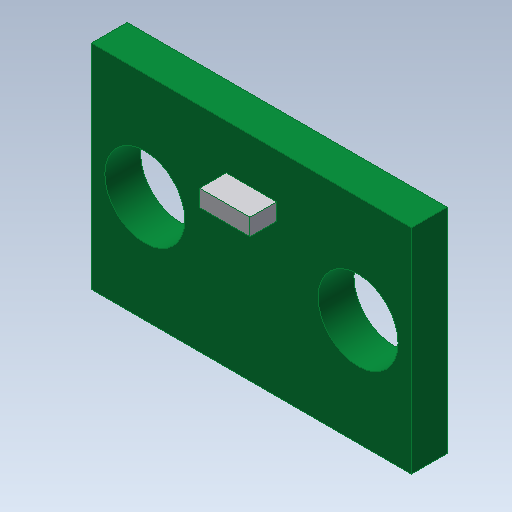
# Autodesk Inventor part: J002609
Saved by Autodesk Inventor 2020.3 (Build 243373000, 373)
## iProperties
RuleStatus: InUse
AfterDocSave0: file://Part Number Cleaner
Created: 2014-07-03
Material: Generic
Vendor: HHMI: JFRC - ID&F
Document SubType Name: Modeling
Designer: NEGRASHOVI
Density: 1 g/cm^3
Part Number: J002609
Appearance: Smooth - Dark Forest Green
DESIGN DEPARTMENT: HHMI: JFRC - ID&F
ALTERED ITEM PART NUMBER: N/A
ALTERED ITEM VENDOR: N/A
ALTERED ITEM DESCRIPTION: N/A
Author: NEGRASHOVI
Revision Number: 0
Autodesk Inventor part; units mm, degrees
ref_plane "YZ Plane" through (0, 0, 0) normal (1, 0, 0) x (0, 1, 0)
ref_plane "XZ Plane" through (0, 0, 0) normal (0, 1, 0) x (-1, 0, 0)
ref_plane "XY Plane" through (0, 0, 0) normal (0, 0, 1) x (1, 0, 0)
sketch "Sketch1" plane through (0, 0, 0) normal (0, 0, 1) x (1, 0, 0)
  line L0 (-7.62, -7.62) -> (7.62, -7.62)
  line L1 (7.62, -7.62) -> (7.62, 2.54)
  line L2 (7.62, 2.54) -> (-7.62, 2.54)
  line L3 (-7.62, 2.54) -> (-7.62, -7.62)
  line L4 (-10.668, 0) -> (10.668, 0) construction
  line L5 (0, -9.652) -> (0, 4.572) construction
  point P0 (0, 0)
  dimension "d0" = 10.16
  dimension "d1" = 15.24
  dimension "d2" = 2.54
  constraints: 8 end point, 2 parallel, 1 horizontal, 1 perpendicular, 1 other
  measures "d0" distance of L2.end L0.start
  measures "d1" distance of L1.end L2.end
  measures "d2" distance between parallel lines of L4 L2
extrude "Extrusion1" add sketch "Sketch1" along normal blind 1.7018
sketch "Sketch2" plane through (0, 0, 1.7018) normal (0, 0, 1) x (1, 0, 0)
  line L0 (-7.62, -7.62) -> (-7.62, 2.54) projected
  line L1 (7.62, -7.62) -> (-7.62, -7.62) projected
  line L2 (7.62, 2.54) -> (7.62, -7.62) projected
  line L3 (-7.62, 2.54) -> (7.62, 2.54) projected
  line L4 (-10.668, 0) -> (10.668, 0) construction
  line L5 (0, -9.652) -> (0, 4.572) construction
  line L6 (-7.62, -2.54) -> (7.62, -2.54) construction
  circle A0 centre (-5.08, -2.54) radius 1.905
  circle A1 centre (5.08, -2.54) radius 1.905
  point P0 (0, 0)
  dimension "d5" = 10.16
  dimension "d6" = 3.81
  constraints: 2 centre point, 2 end point, 2 midpoint, 2 point on line, 1 equal radius, 1 other
  measures "d5" distance of A1.centre A0.centre
  measures "d6" diameter of A0
extrude "Extrusion2" cut sketch "Sketch2" against normal through all contours A0 | A1
sketch "Sketch3" plane through (0, 0, 1.7018) normal (0, 0, 1) x (1, 0, 0)
  line L0 (-10.668, 0) -> (10.668, 0) construction
  line L1 (0, -9.652) -> (0, 4.572) construction
  line L2 (-1.2001, 0.4) -> (1.2002, 0.4001)
  line L3 (1.2002, 0.4001) -> (1.2002, -0.4001)
  line L4 (1.2002, -0.4001) -> (-1.2001, -0.4)
  line L5 (-1.2001, -0.4) -> (-1.2001, 0.4)
  point P0 (0, 0)
  dimension "d9" = 0.8001
  dimension "d10" = 2.4003
  constraints: 8 end point, 2 parallel, 1 horizontal, 1 perpendicular, 2 other
  measures "d9" distance of L2.end L3.end
  measures "d10" distance of L2.start L2.end
extrude "Extrusion3" add sketch "Sketch3" along normal blind 1.27
sketch "Sketch4" plane through (0, 0, 0) normal (0, 0, -1) x (-1, 0, 0)
  circle A0 centre (2.54, 0.1778) radius 0.635 projected
  circle A1 centre (0, 0.1778) radius 0.635 projected
  circle A2 centre (-2.54, 0.1778) radius 0.635 projected
  point P0 (0, 0)
body "Solid1"
